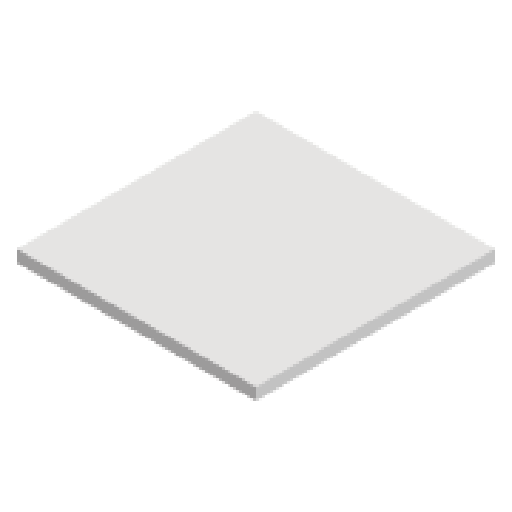
# Autodesk Inventor part: 00_Polfilter_rectangular_20mm
Saved by Autodesk Inventor 2025.1 (Build 291241020, 241B)
## iProperties
Created: 2024-10-07
Part Number: 00_Polfilter_rectangular_20mm
Material: Generic
Document SubType Name: Modeling
Designer: diederichbenedict
Density: 1 g/cm^3
Appearance: Default
Author: diederichbenedict
Autodesk Inventor part; units mm, degrees
ref_plane "YZ Plane" through (0, 0, 0) normal (1, 0, 0) x (0, 1, 0)
ref_plane "XZ Plane" through (0, 0, 0) normal (0, 1, 0) x (-1, 0, 0)
ref_plane "XY Plane" through (0, 0, 0) normal (0, 0, 1) x (1, 0, 0)
sketch "Sketch1" plane through (0, 0, 0) normal (0, 0, 1) x (1, 0, 0)
  line L0 (10, -10) -> (-10, -10)
  line L1 (-10, -10) -> (-10, 10)
  line L2 (-10, 10) -> (10, 10)
  line L3 (10, 10) -> (10, -10)
  line L4 (10, -10) -> (-10, 10) construction
  line L5 (-10, -10) -> (10, 10) construction
  point P0 (0, 0)
  dimension "d0" = 20
  dimension "d1" = 20
  constraints: 12 end point, 2 midpoint, 2 parallel, 1 horizontal, 1 perpendicular
  measures "d0" distance of L1.end L2.end
  measures "d1" distance of L0.end L1.end
extrude "Extrusion1" add sketch "Sketch1" along normal blind 1
body "Solid1"
